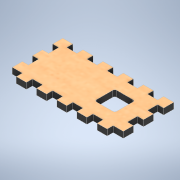
# Autodesk Inventor part: plate_front_small
Saved by Autodesk Inventor 2021 (Build 250183000, 183)
## iProperties
Created: 2021-03-07
Part Number: plate_front_small
Material: Holz (Kirsche)
Document SubType Name: Modeling
Designer: Tilman
Density: 0.63 g/cm^3
Appearance: Glänzend - Schwarz
Author: Tilman
Autodesk Inventor part; units mm, degrees
ref_plane "YZ Plane" through (0, 0, 0) normal (1, 0, 0) x (0, 1, 0)
ref_plane "XZ Plane" through (0, 0, 0) normal (0, 1, 0) x (-1, 0, 0)
ref_plane "XY Plane" through (0, 0, 0) normal (0, 0, 1) x (1, 0, 0)
sketch "Skizze1" plane through (0, 0, 0) normal (0, 1, 0) x (-1, 0, 0)
  line L0 (-5, 0) -> (-5, -3)
  line L1 (-5, -3) -> (0, -3)
  line L2 (-5, 0) -> (-10, 0)
  line L3 (-10, 0) -> (-10, -3)
  line L4 (-10, -3) -> (-15, -3)
  line L5 (-15, 0) -> (-15, -3)
  line L6 (-15, 0) -> (-20, 0)
  line L7 (-20, 0) -> (-20, -3)
  line L8 (-20, -3) -> (-25, -3)
  line L9 (-25, 0) -> (-25, -3)
  line L10 (-25, 0) -> (-30, 0)
  line L11 (-30, 0) -> (-30, -3)
  line L12 (-30, -3) -> (-35, -3)
  line L13 (-35, 0) -> (-35, -3)
  line L14 (-35, 0) -> (-40, 0)
  line L15 (-40, 0) -> (-40, -3)
  line L16 (-40, -3) -> (-45, -3)
  line L17 (-45, 0) -> (-45, -3)
  line L18 (-45, 0) -> (-50, 0)
  line L19 (-50, 0) -> (-50, -3)
  line L20 (-50, -3) -> (-55, -3)
  line L21 (-55, -3) -> (-55, -8)
  line L22 (-55, -8) -> (-52, -8)
  line L23 (-52, -8) -> (-52, -13)
  line L24 (-52, -13) -> (-55, -13)
  line L25 (0, -3) -> (0, -8)
  line L26 (0, -8) -> (-3, -8)
  line L27 (-3, -8) -> (-3, -13)
  line L28 (-3, -13) -> (0, -13)
  line L29 (-52, -18) -> (-52, -23)
  line L30 (-55, -13) -> (-55, -18)
  line L31 (-52, -23) -> (-55, -23)
  line L32 (-55, -18) -> (-52, -18)
  line L33 (-3, -18) -> (-3, -23)
  line L34 (-3, -23) -> (0, -23)
  line L35 (0, -18) -> (-3, -18)
  line L36 (0, -13) -> (0, -18)
  line L37 (0, -23) -> (0, -28)
  line L38 (0, -28) -> (-5, -28)
  line L39 (-5, -28) -> (-5, -25)
  line L40 (-5, -25) -> (-10, -25)
  line L41 (-10, -25) -> (-10, -28)
  line L42 (-55, -23) -> (-55, -28)
  line L43 (-15, -25) -> (-20, -25)
  line L44 (-20, -25) -> (-20, -28)
  line L45 (-10, -28) -> (-15, -28)
  line L46 (-15, -28) -> (-15, -25)
  line L47 (-25, -25) -> (-30, -25)
  line L48 (-30, -25) -> (-30, -28)
  line L49 (-20, -28) -> (-25, -28)
  line L50 (-25, -28) -> (-25, -25)
  line L51 (-35, -25) -> (-40, -25)
  line L52 (-40, -25) -> (-40, -28)
  line L53 (-30, -28) -> (-35, -28)
  line L54 (-35, -28) -> (-35, -25)
  line L55 (-45, -25) -> (-50, -25)
  line L56 (-50, -25) -> (-50, -28)
  line L57 (-40, -28) -> (-45, -28)
  line L58 (-45, -28) -> (-45, -25)
  line L59 (-50, -28) -> (-55, -28)
  line L60 (-35.75, -19) -> (-43.75, -19)
  line L61 (-44.75, -18) -> (-44.75, -10)
  line L62 (-43.75, -9) -> (-35.75, -9)
  line L63 (-34.75, -10) -> (-34.75, -18)
  arc A0 (-35.75, -19) -> (-34.75, -18) centre (-35.75, -18) ccw
  arc A1 (-44.75, -18) -> (-43.75, -19) centre (-43.75, -18) ccw
  arc A2 (-43.75, -9) -> (-44.75, -10) centre (-43.75, -10) ccw
  arc A3 (-34.75, -10) -> (-35.75, -9) centre (-35.75, -10) ccw
  line L64 (-27.5, -28) -> (-27.5, 0) construction
  line L65 (-27.5, -14) -> (-52, -14) construction
  point P0 (0, 0)
  point P1 (-34.75, -14)
  point P2 (-39.75, -14)
  point P3 (-39.75, -19)
  dimension "d2" = 5
  dimension "d3" = 3
  dimension "d6" = 10
  dimension "d22" = 10
  dimension "d29" = 10
  dimension "d34" = 1
  dimension "d36" = 10
  dimension "d37" = 10
  constraints: 132 end point, 14 equal length, 13 perpendicular, 9 point on line, 9 vertical, 8 point on circle, 8 tangent, 7 horizontal, 5 midpoint, 4 centre point, 3 collinear, 3 equal radius, 3 horizontal alignment, 3 vertical alignment, 87 other
  measures "d2" distance of L0.start L2.end
  measures "d3" distance of L0.start L0.end
  measures "d6" distance of L0.start L5.start
  measures "d22" distance of L22.end L29.start
  measures "d29" distance of L40.end L43.end
  measures "d34" radius of A0
  measures "d36" distance between parallel lines of L61 L63
  measures "d37" distance between parallel lines of L62 L60
extrude "Extrusion1" add sketch "Skizze1" along normal blind 3
